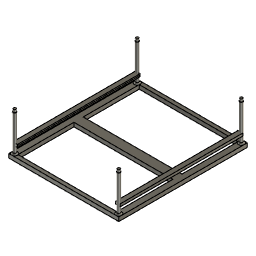
box_support (Autodesk Fusion 360 design; units mm, degrees)
Autodesk Fusion 360 part; units mm, degrees
sketch "sk_base" plane through (0, 0, 0) normal (0, 0, 1) x (1, 0, 0)
  line L0 (77, 91) -> (-77, 91)
  line L1 (-77, 91) -> (-77, -91)
  line L2 (-77, -91) -> (77, -91)
  line L3 (77, -91) -> (77, 91)
  line L4 (77, 91) -> (-77, -91) construction
  line L5 (-77, 91) -> (77, -91) construction
  line L6 (-83.5, -97.5) -> (83.5, -97.5)
  line L7 (83.5, -97.5) -> (83.5, 97.5)
  line L8 (83.5, 97.5) -> (-83.5, 97.5)
  line L9 (-83.5, 97.5) -> (-83.5, -97.5)
  circle A0 centre (-79, 93) radius 2.5
  circle A1 centre (79, 93) radius 2.5
  circle A2 centre (-79, -93) radius 2.5
  circle A3 centre (79, -93) radius 2.5
  dimension "d1" = 154
  dimension "d2" = 182
  dimension "d3" = 6.5
  dimension "d4" = 5
  dimension "d5" = 5
  dimension "d6" = 5
  dimension "d7" = 5
  constraint horizontal L0
  constraint perpendicular L0 L1
  constraint parallel L0 L2
  constraint parallel L1 L3
  constraint coincident L4 origin
  constraint coincident L5 origin
  measures "d1" distance of L1.end L2.end
  measures "d2" distance of L0.end L1.end
  measures "d4" diameter of A0
  measures "d5" diameter of A1
  measures "d6" diameter of A2
  measures "d7" diameter of A3
extrude "Extrude2" add sketch "sk_base" against normal blind 6 contours L0 L1 L2 L3 | L6 L7 L8 L9 makes body 1
extrude "Extrude1" add sketch "sk_base" along normal blind 55 separate body contours A0 | A1 | A2 | A3 makes body 2 at (-76.5124, -93.2489, 18.3333) makes body 3 at (76.6963, -93.9711, 36.6667) makes body 4 at (-81.3037, 92.0289, 36.6667) makes body 5 at (76.6963, 92.0289, 36.6667)
sketch "sk_rail" plane through (-83.5, 0, 0) normal (-1, 0, 0) x (0, -1, 0)
  line L0 (97.5, 0) -> (-97.5, 0)
  line L1 (-97.5, 0) -> (-97.5, -6)
  line L2 (-97.5, -6) -> (97.5, -6)
  line L3 (97.5, -6) -> (97.5, 0)
  line L4 (-92.7862, 10.2075) -> (93.2138, 10.2075)
  line L5 (93.2138, 10.2075) -> (93.2138, 14.2075)
  line L6 (93.2138, 14.2075) -> (-92.7862, 14.2075)
  line L7 (-92.7862, 14.2075) -> (-92.7862, 10.2075)
  dimension "d12" = 186
  dimension "d13" = 4
  constraint horizontal L4
  constraint vertical L5
  constraint horizontal L6
  constraint vertical L7
  measures "d12" distance of L4.start L4.end
  measures "d13" distance of L4.start L6.end
extrude "Extrude3" add sketch "sk_rail" against normal blind 10 separate body contours L4 L5 L6 L7 makes body 6
extrude "Extrude4" cut 1 faces at (-83.5, -31.2138, 12.8742) along direction (1, 0, 0) blind 2 on bodies 6 bodies 6
fillet "Fillet1" radius 1 4 edges at (-73.5, -0.2138, 14.2075) (-73.5, -93.2138, 12.2075) (-73.5, -0.2138, 10.2075) (-73.5, 92.7862, 12.2075) on bodies 6
mirror "Mirror1" about plane through (0, 0, 0) normal (1, 0, 0) of bodies 6 makes body 7
box "BoxPrimitive1" cut length 85 width 150 height -15 placed x (0, 1, 0) y (-1, 0, 0) z (0, 0, 1) at (75, 7, 0) bodies 1
mirror "Mirror2" about plane through (0, 0, 0) normal (0, 1, 0) of "BoxPrimitive1"
extrude "Extrude5" add sketch "sk_base" against normal blind 1 contours A1 bodies 1 7 5
extrude "Extrude6" add sketch "sk_base" against normal blind 1 contours A3 bodies 1 7 3
extrude "Extrude7" add sketch "sk_base" against normal blind 1 contours A2 bodies 1 6 2
extrude "Extrude8" add sketch "sk_base" against normal blind 1 contours A0 bodies 1 6 4
fillet "Fillet2" radius 2 4 edges at (-81.3308, 93.904, 0) (-81.3308, -92.096, 0) (76.6692, -92.096, 0) (76.6692, 93.904, 0) on bodies 1
sketch "sk_foot_ext_1" plane through (0, 0, 55) normal (0, 0, 1) x (-1, 0, 0)
  circle A0 centre (-79, 93) radius 2.5
  circle A1 centre (-79, 93) radius 2
  constraint concentric A0 A1
extrude "Extrude9" add sketch "sk_foot_ext_1" along normal blind 4 contours A1 bodies 1
sketch "sk_foot_ext_2" plane through (0, 0, 55) normal (0, 0, 1) x (-1, 0, 0)
  circle A0 centre (79, 93) radius 2.5
  circle A1 centre (79, 93) radius 2
  constraint concentric A0 A1
extrude "Extrude10" add sketch "sk_foot_ext_2" along normal blind 4 contours A1 bodies 1
sketch "sk_foot_ext_3" plane through (0, 0, 55) normal (0, 0, 1) x (-1, 0, 0)
  circle A0 centre (79, -93) radius 2.5
  circle A1 centre (79, -93) radius 2
  dimension "d43" = 4
  constraint concentric A0 A1
  measures "d43" diameter of A1
extrude "Extrude11" add sketch "sk_foot_ext_3" along normal blind 4 contours A1 bodies 1
sketch "sk_foot_ext_4" plane through (0, 0, 55) normal (0, 0, 1) x (-1, 0, 0)
  circle A0 centre (-79, -93) radius 2.5
  circle A1 centre (-79, -93) radius 2
  dimension "d46" = 4
  constraint concentric A0 A1
  measures "d46" diameter of A1
extrude "Extrude12" add sketch "sk_foot_ext_4" along normal blind 4 contours A1 bodies 1
extrude "Extrude13" add 1 faces at (80.7603, -93.1944, -1) along direction (0, 0, -1) blind 1 on bodies 1 bodies 1
extrude "Extrude14" add 1 faces at (-77.2397, -93.1944, -1) along direction (0, 0, -1) blind 1 on bodies 1 bodies 1
extrude "Extrude15" add 1 faces at (-77.2397, 92.8056, -1) along direction (0, 0, -1) blind 1 on bodies 1 bodies 1
extrude "Extrude16" add 1 faces at (77.2397, 92.8056, -1) along direction (0, 0, -1) blind 1 on bodies 1 bodies 1
named bodies: "b_foot_front_right", "b_foot_front_left", "b_foot_back_right", "b_foot_back_left", "b_base", "b_rail_right", "b_rail_left"
